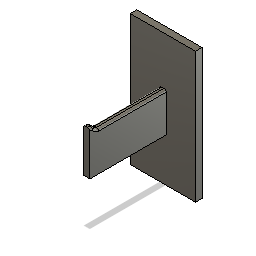
GHD Stand v2 (Autodesk Fusion 360 design; units mm, degrees)
Autodesk Fusion 360 part; units mm, degrees
sketch "Sketch1" plane through (0, 0, 0) normal (0, 0, 1) x (1, 0, 0)
  line L0 (15, 30) -> (-15, 30)
  line L1 (-15, 30) -> (-15, -30)
  line L2 (-15, -30) -> (15, -30)
  line L3 (15, -30) -> (15, 30)
  line L4 (15, 30) -> (-15, -30) construction
  line L5 (-15, 30) -> (15, -30) construction
  line L6 (1.5, 10) -> (-1.5, 10)
  line L7 (-1.5, 10) -> (-1.5, -10)
  line L8 (-1.5, -10) -> (1.5, -10)
  line L9 (1.5, -10) -> (1.5, 10)
  line L10 (1.5, 10) -> (-1.5, -10) construction
  line L11 (-1.5, 10) -> (1.5, -10) construction
  dimension "d1" = 60
  dimension "d2" = 30
  dimension "d3" = 20
  dimension "d4" = 3
  constraint perpendicular L0 L1
  constraint parallel L0 L2
  constraint parallel L1 L3
  constraint horizontal L0
  constraint coincident L4 origin
  constraint coincident L5 origin
  constraint perpendicular L6 L7
  constraint parallel L6 L8
  constraint parallel L7 L9
  constraint horizontal L6
  constraint coincident L10 origin
  constraint coincident L11 origin
  measures "d1" distance of L0.start L2.end
  measures "d2" distance of L0.start L0.end
  measures "d3" distance of L6.start L8.end
  measures "d4" distance of L7.end L8.end
extrude "Extrude1" add sketch "Sketch1" against normal blind 3 contours L0 L1 L2 L3 | L6 L7 L8 L9
extrude "Extrude2" add sketch "Sketch1" along normal blind 35 contours L6 L7 L8 L9
sketch "Sketch2" plane through (0, 0, 0) normal (1, 0, 0) x (0, 0, -1)
sketch "Sketch3" plane through (1.5, 0, 0) normal (1, 0, 0) x (0, 0, -1)
  line L0 (0, -10) -> (0, 10)
  line L1 (0, 10) -> (-35, 10)
  line L2 (-35, 10) -> (-35, -10)
  line L3 (-35, -10) -> (0, -10)
  line L4 (0, 10) -> (-33, 10)
  line L5 (-33, 10) -> (-33, 8) construction
  line L6 (-33, 8) -> (0, 8)
  line L7 (0, 8) -> (0, 10)
  arc A0 (-33, 10) -> (-31, 8) centre (-31, 10) ccw
  dimension "d9" = 2
  dimension "d10" = 33
  dimension "d15" = 4
  constraint horizontal L4
  constraint vertical L5
  constraint horizontal L6
  constraint vertical L7
  constraint coincident L0.end L1.start
  constraint tangent L5 A0
  constraint tangent L6 A0
  constraint coincident L6 A0.end
  measures "d9" distance of L4.end L5.end
  measures "d10" distance of L5.end L6.end
  measures "d15" diameter of A0
extrude "Extrude3" cut sketch "Sketch3" against normal through all contours L0 L1 L4 L6 L7 A0
fillet "Fillet4" radius 1 2 edges at (1.5, 8, 15.5) (1.5, 8.5858, 32.4142)
fillet "Fillet5" radius 1 2 edges at (-1.5, 8.5858, 32.4142) (-1.5, 8, 15.5)
fillet "Fillet6" radius 1 5 edges at (-1.5, 10, 34.5) (-1.2071, 10, 33.2929) (0, 10, 33) (1.2071, 10, 33.2929) (1.5, 10, 34.5)
